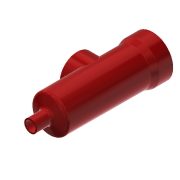
# Autodesk Inventor part: 01_Connector_T
Saved by Autodesk Inventor 2019.4 (Build 234330000, 330)
## iProperties
Created: 2021-06-01
Part Number: 01_Connector_T
Material: Generic
Document SubType Name: Modeling
Designer: diederichbenedict
Density: 1 g/cm^3
Appearance: Smooth - Red
Author: diederichbenedict
Autodesk Inventor part; units mm, degrees
ref_plane "YZ Plane" through (0, 0, 0) normal (1, 0, 0) x (0, 1, 0)
ref_plane "XZ Plane" through (0, 0, 0) normal (0, 1, 0) x (-1, 0, 0)
ref_plane "XY Plane" through (0, 0, 0) normal (0, 0, 1) x (1, 0, 0)
sketch "Sketch1" plane through (0, 0, 0) normal (1, 0, 0) x (0, 1, 0)
  line L0 (11, 0) -> (11, -20)
  line L1 (-11, 0) -> (11, 0)
  line L2 (13, -15.30202) -> (0, -15.30202)
  line L3 (0, -15.30202) -> (0, 51.69798)
  line L4 (0, 51.69798) -> (4, 51.69798)
  line L5 (4, 51.69798) -> (11, 0) construction
  line L6 (4, 51.69798) -> (11.638351, 49.69798)
  line L7 (11.638351, 49.69798) -> (11.638351, 44.69798)
  line L8 (4, 51.69798) -> (0, 51.69798)
  line L9 (0, 51.69798) -> (0, 61.69798)
  line L10 (0, 61.69798) -> (4, 61.69798)
  line L11 (4, 61.69798) -> (4, 51.69798)
  line L12 (-11.938351, 38.617239) -> (11.938351, 38.617239)
  line L13 (11.638351, 44.69798) -> (11.638351, -2.697214)
  line L14 (11.638351, -2.697214) -> (13, -6.743325)
  line L15 (13, -6.743325) -> (13, -15.30202)
  point P0 (0, 0)
  point P1 (9.115, 0)
  dimension "d12" = 4
  dimension "d13" = 0
  dimension "d15" = 13
  dimension "d17" = 2
  dimension "d19" = 5
  dimension "d20" = 10
  dimension "d25" = 65
  dimension "d26" = 0.3
  constraints: 30 end point, 4 parallel, 3 horizontal, 3 perpendicular, 2 point on line, 1 vertical, 4 other
  measures "d12" distance between parallel lines of L11 L9
  measures "d13" distance from line of point (0, 0) L3
  measures "d15" distance of L2.end L2.start
  measures "d17" distance from line of L6.end L4
  measures "d19" distance of L7.end L6.end
  measures "d20" distance between parallel lines of L4 L10
  measures "d25" distance from line of L2 L6.end
  measures "d26" distance from line of L12.end L13
revolve "Revolution1" add sketch "Sketch1" angle 360 about axis through (0, 0, -15.30202) along (0, 0, 1)
sketch "Sketch5" plane through (0, 0, 0) normal (1, 0, 0) x (0, 1, 0)
  circle A0 centre (0, 17.334358) radius 7.78
  circle A1 centre (0, 17.334358) radius 10.974581
  circle A2 centre (0, 17.334358) radius 7.78
  point P0 (0, 0)
  constraints: 3 centre point, 1 coincident, 4 other
extrude "Extrusion3" add sketch "Sketch5" against normal blind 15 contours A0 | A1
sketch "Sketch6" plane through (-15, 0, 17.334358) normal (-1, 0, 0) x (0, 0, 1)
  circle A0 centre (0, 0) radius 7.78
  circle A1 centre (0, 0) radius 8.043974
  point P0 (-17.334358, 0)
  constraints: 2 centre point, 1 coincident, 2 other
sketch "Sketch6 outline for Extrusion4" plane through (-15, 0, 17.334358) normal (-1, 0, 0) x (0, 0, 1)
  circle A0 centre (0, 0) radius 8.043974
extrude "Extrusion4" cut sketch "Sketch6 outline for Extrusion4" against normal blind 15 draft -4
sketch "Sketch7" plane through (0, 0, 0) normal (0, 1, 0) x (-1, 0, 0)
  point P0 (0, 0)
fillet "Fillet2" radius 2 2 edges at (0, -4, 51.698) (0, -11.6384, 49.698)
sketch "Sketch4" plane through (0, 0, 61.69798) normal (0, 0, 1) x (1, 0, 0)
  circle A0 centre (0, 0) radius 1.479649
  circle A1 centre (0, 0) radius 4
  circle A2 centre (0, 0) radius 3.2
  point P0 (0, 0)
  dimension "d21" = 6.4
  constraints: 1 centre point, 1 coincident
  measures "d21" diameter of A2
extrude "Extrusion2" cut sketch "Sketch4" against normal through all contours A0 | A2
sketch "Sketch8" plane through (0, 0, -15.30202) normal (0, 0, -1) x (-1, 0, 0)
  circle A0 centre (0, 0) radius 11.2
  point P0 (0, 0)
  constraints: 1 centre point, 2 other
extrude "Extrusion5" cut sketch "Sketch8" against normal blind 65 draft -2
fillet "Fillet3" radius 2 6 edges at (-6.7477, -7.4663, 17.2395) (-6.7477, 7.4663, 17.2394) (8.9301, 0, 49.698) (-3.2, 0, 49.698) (0, -11.6384, -2.6972) (0, -13, -6.7433)
body "Solid1"
